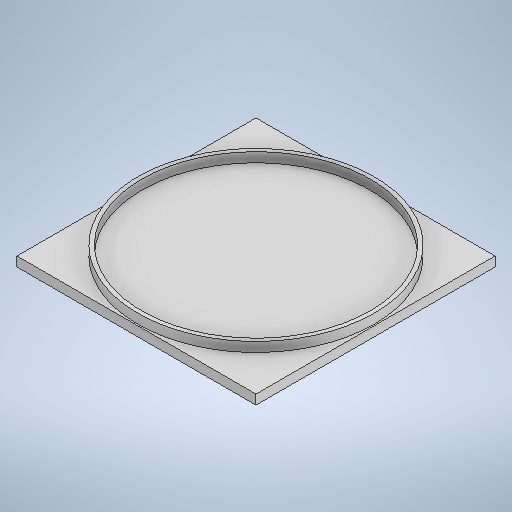
# Autodesk Inventor part: dot_antirol
Saved by Autodesk Inventor 2025.1 (Build 291241000, 241)
## iProperties
Created: 2025-05-15
Part Number: dot_antirol
Material: Generic
Document SubType Name: Modeling
Designer: santiago
Density: 1 g/cm^3
Appearance: Default
Author: santiago
Autodesk Inventor part; units mm, degrees
ref_plane "YZ Plane" through (0, 0, 0) normal (1, 0, 0) x (0, 1, 0)
ref_plane "XZ Plane" through (0, 0, 0) normal (0, 1, 0) x (-1, 0, 0)
ref_plane "XY Plane" through (0, 0, 0) normal (0, 0, 1) x (1, 0, 0)
sketch "Sketch1" plane through (0, 0, 0) normal (0, 1, 0) x (-1, 0, 0)
  line L0 (7.5, -7.5) -> (-7.5, -7.5)
  line L1 (-7.5, -7.5) -> (-7.5, 7.5)
  line L2 (-7.5, 7.5) -> (7.5, 7.5)
  line L3 (7.5, 7.5) -> (7.5, -7.5)
  line L4 (7.5, -7.5) -> (-7.5, 7.5) construction
  line L5 (-7.5, -7.5) -> (7.5, 7.5) construction
  point P0 (0, 0)
  dimension "d0" = 15
  dimension "d1" = 15
  constraints: 12 end point, 2 midpoint, 2 parallel, 1 horizontal, 1 perpendicular
  measures "d0" distance of L1.end L2.end
  measures "d1" distance of L0.end L1.end
extrude "Extrusion1" add sketch "Sketch1" along normal blind 0.6
sketch "Sketch2" plane through (0, 0.6, 0) normal (0, 1, 0) x (1, 0, 0)
  circle A0 centre (0, 0) radius 7.165
  circle A1 centre (0, 0) radius 7.415
  dimension "d4" = 14.33
  dimension "d5" = 14.83
  constraints: 2 centre point, 2 coincident
  measures "d4" diameter of A0
  measures "d5" diameter of A1
extrude "Extrusion2" add sketch "Sketch2" along normal blind 0.6
equation "\"d1\" = d0"
body "Solid1"
